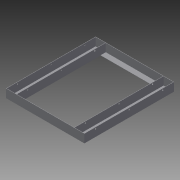
# Autodesk Inventor part: Base
Saved by Autodesk Inventor 2015 (Build 190159000, 159)
## iProperties
Created: 2015-01-10
Part Number: Base
Material: Generic
Document SubType Name: Modeling
Designer: Chandler Willoughby
Density: 1 g/cm^3
Appearance: Default
Author: Chandler Willoughby
Autodesk Inventor part; units mm, degrees
ref_plane "YZ Plane" through (0, 0, 0) normal (1, 0, 0) x (0, 1, 0)
ref_plane "XZ Plane" through (0, 0, 0) normal (0, 1, 0) x (-1, 0, 0)
ref_plane "XY Plane" through (0, 0, 0) normal (0, 0, 1) x (1, 0, 0)
sketch "Sketch1" plane through (0, 0, 0) normal (0, 1, 0) x (-1, 0, 0)
  line L0 (0, 0) -> (711.2, 0)
  line L1 (711.2, 0) -> (711.2, -812.8)
  line L2 (711.2, -812.8) -> (0, -812.8)
  line L3 (0, -812.8) -> (0, 0)
  line L4 (0, 0) -> (711.2, 0)
  line L5 (711.2, 0) -> (711.2, -76.2)
  line L6 (0, -76.2) -> (0, 0)
  line L7 (0, -812.8) -> (711.2, -812.8)
  line L8 (711.2, -812.8) -> (711.2, -736.6)
  line L9 (0, -736.6) -> (0, -812.8)
  line L10 (0, 0) -> (25.4, 0)
  line L11 (25.4, -76.2) -> (25.4, -736.6)
  line L12 (25.4, -812.8) -> (0, -812.8)
  line L13 (0, -812.8) -> (0, 0)
  line L14 (711.2, 0) -> (685.8, 0)
  line L15 (685.8, -76.2) -> (685.8, -736.6)
  line L16 (685.8, -812.8) -> (711.2, -812.8)
  line L17 (711.2, -812.8) -> (711.2, 0)
  line L18 (685.8, -736.6) -> (635, -736.6)
  line L19 (615.95, -736.6) -> (615.95, -76.2)
  line L20 (635, -76.2) -> (635, -736.6)
  line L21 (25.4, -736.6) -> (76.2, -736.6)
  line L22 (95.25, -736.6) -> (95.25, -76.2)
  line L23 (76.2, -76.2) -> (76.2, -736.6)
  line L24 (685.8, -76.2) -> (635, -76.2)
  line L25 (685.8, -736.6) -> (635, -736.6)
  line L26 (615.95, -736.6) -> (95.25, -736.6)
  line L27 (76.2, -736.6) -> (25.4, -736.6)
  line L28 (615.95, -76.2) -> (95.25, -76.2)
  line L29 (76.2, -76.2) -> (25.4, -76.2)
  dimension "d0" = 711.2
  dimension "d1" = 812.8
  dimension "d2" = 76.2
  dimension "d3" = 76.2
  dimension "d4" = 25.4
  dimension "d5" = 25.4
  dimension "d6" = 812.8
  dimension "d10" = 660.4
  constraints: 60 end point, 16 parallel, 5 horizontal, 5 perpendicular, 3 point on line
  measures "d0" distance of L1.end L2.end
  measures "d1" distance of L0.end L1.end
  measures "d2" distance of L4.end L5.end
  measures "d3" distance of L8.end L7.end
  measures "d4" distance of L12.start L12.end
  measures "d5" distance of L16.end L16.start
  measures "d6" distance of L16.start L14.end
  measures "d10" distance of L19.start L19.end
extrude "Extrusion1" add sketch "Sketch1" along normal blind 3.175
sketch "Sketch2" plane through (0, 3.175, 0) normal (0, 1, 0) x (1, 0, 0)
  line L0 (-711.2, 812.8) -> (0, 812.8)
  line L1 (0, 812.8) -> (0, 0)
  line L2 (0, 0) -> (-711.2, 0)
  line L3 (-711.2, 0) -> (-711.2, 812.8)
  line L4 (-708.025, 809.625) -> (-3.175, 809.625)
  line L5 (-3.175, 809.625) -> (-3.175, 3.175)
  line L6 (-3.175, 3.175) -> (-708.025, 3.175)
  line L7 (-708.025, 3.175) -> (-708.025, 809.625)
  constraints: 16 end point, 4 parallel, 2 horizontal, 2 perpendicular
extrude "Extrusion2" add sketch "Sketch2" along normal blind 73.025
sketch "Sketch3" plane through (0, 0, 0) normal (0, -1, 0) x (1, 0, 0)
  line L0 (-25.4, -76.2) -> (-25.4, -50.8)
  line L1 (-25.4, -50.8) -> (-685.8, -50.8)
  line L2 (-685.8, -50.8) -> (-685.8, -762)
  line L3 (-685.8, -762) -> (-25.4, -762)
  line L4 (-25.4, -762) -> (-25.4, -50.8)
  line L5 (-25.4, -76.2) -> (-76.2, -76.2)
  line L6 (-76.2, -76.2) -> (-76.2, -50.8)
  line L7 (-95.25, -76.2) -> (-95.25, -50.8)
  line L8 (-95.25, -76.2) -> (-615.95, -76.2)
  line L9 (-615.95, -76.2) -> (-615.95, -50.8)
  line L10 (-635, -76.2) -> (-635, -50.8)
  line L11 (-635, -76.2) -> (-685.8, -76.2)
  line L12 (-95.25, -736.6) -> (-95.25, -762)
  line L13 (-95.25, -736.6) -> (-615.95, -736.6)
  line L14 (-615.95, -736.6) -> (-615.95, -762)
  line L15 (-635, -736.6) -> (-635, -762)
  line L16 (-635, -736.6) -> (-685.8, -736.6)
  line L17 (-635, -50.8) -> (-685.8, -50.8)
  line L18 (-685.8, -50.8) -> (-685.8, -76.2)
  line L19 (-685.8, -736.6) -> (-685.8, -762)
  line L20 (-685.8, -762) -> (-635, -762)
  line L21 (-615.95, -762) -> (-95.25, -762)
  line L22 (-95.25, -762) -> (-95.25, -736.6)
  line L23 (-25.4, -736.6) -> (-25.4, -76.2) projected
  line L24 (-25.4, -762) -> (-76.2, -762)
  line L25 (-76.2, -762) -> (-76.2, -736.6)
  line L26 (-76.2, -736.6) -> (-25.4, -736.6)
  line L27 (-25.4, -736.6) -> (-25.4, -762)
  point P0 (0, 0)
  dimension "d22" = 25.4
  dimension "d23" = 660.4
  dimension "d24" = 711.2
  dimension "d25" = 25.4
  dimension "d26" = 25.4
  constraints: 54 end point, 12 perpendicular, 8 point on line, 6 horizontal, 2 collinear, 2 parallel, 1 vertical
  measures "d22" distance of L0.start L0.end
  measures "d23" distance of L0.end L1.end
  measures "d24" distance of L1.end L2.end
  measures "d25" distance of L8.end L9.end
  measures "d26" distance of L13.end L14.end
extrude "Extrusion3" cut sketch "Sketch3" against normal blind 73.025 contours L5 L6 L1 L0 | L4 L3 L25 L26 | L7 L8 L9 L1 | L3 L14 L13 L12 | L10 L11 L2 L1 | L3 L2 L16 L15
sketch "Sketch4" plane through (-711.2, 0, -812.8) normal (-1, 0, 0) x (0, 0, 1)
  line L0 (812.8, 76.2) -> (406.4, 76.2)
  line L1 (812.8, 76.2) -> (0, 76.2) projected
  line L2 (762, 0) -> (50.8, 0) projected
  circle A0 centre (406.4, 63.5) radius 6.35
  circle A1 centre (711.2, 63.5) radius 6.35
  circle A2 centre (101.6, 63.5) radius 6.35
  point P0 (812.8, 0)
  dimension "d29" = 406.4
  dimension "d31" = 12.7
  dimension "d35" = 12.7
  dimension "d36" = 12.7
  constraints: 3 centre point, 2 end point, 1 midpoint
  measures "d29" distance of L0.start L0.end
  measures "d31" diameter of A0
  measures "d35" diameter of A1
  measures "d36" diameter of A2
sketch "Sketch5" plane through (0, 3.175, 0) normal (0, 1, 0) x (1, 0, 0)
  line L0 (-708.025, 3.175) -> (-3.175, 3.175) projected
  line L1 (-3.175, 809.625) -> (-708.025, 809.625) projected
  line L2 (-615.95, 3.175) -> (-619.125, 3.175)
  line L3 (-619.125, 3.175) -> (-619.125, 809.625)
  line L4 (-619.125, 809.625) -> (-615.95, 809.625)
  line L5 (-615.95, 809.625) -> (-615.95, 3.175)
  line L6 (-95.25, 809.625) -> (-92.075, 809.625)
  line L7 (-92.075, 809.625) -> (-92.075, 3.175)
  line L8 (-92.075, 3.175) -> (-95.25, 3.175)
  line L9 (-95.25, 3.175) -> (-95.25, 809.625)
  point P0 (0, 0)
  dimension "d37" = 3.175
  dimension "d38" = 3.175
  constraints: 16 end point, 4 parallel, 4 point on line, 2 horizontal, 2 perpendicular
  measures "d37" distance of L3.end L4.end
  measures "d38" distance of L7.end L8.end
extrude "Extrusion4" add sketch "Sketch5" along normal blind 73.025 contours L3 L1 L5 L0 | L9 L1 L7 L0
extrude "Extrusion5" cut sketch "Sketch4" against normal blind 1016
body "Solid1"
